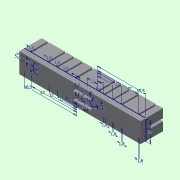
# Autodesk Inventor part: Distance_test_rig
Saved by Autodesk Inventor 2015 (Build 190159000, 159)
## iProperties
Created: 2015-05-18
Part Number: Distance_test_rig
Material: Generic
Document SubType Name: Modeling
Designer: Openlab
Density: 1 g/cm^3
Appearance: Default
Author: Openlab
Autodesk Inventor part; units mm, degrees
ref_plane "YZ Plane" through (0, 0, 0) normal (1, 0, 0) x (0, 1, 0)
ref_plane "XZ Plane" through (0, 0, 0) normal (0, 1, 0) x (-1, 0, 0)
ref_plane "XY Plane" through (0, 0, 0) normal (0, 0, 1) x (1, 0, 0)
sketch "Sketch1" plane through (0, 0, 0) normal (0, 1, 0) x (-1, 0, 0)
  line L0 (73.75, -5.25) -> (61.25, -5.25)
  line L1 (61.25, -5.25) -> (61.25, -17.75)
  line L2 (61.25, -17.75) -> (73.75, -17.75)
  line L3 (73.75, -17.75) -> (73.75, -5.25)
  line L4 (140, 0) -> (0, 0)
  line L5 (0, 0) -> (0, -23)
  line L6 (0, -23) -> (140, -23)
  line L7 (140, -23) -> (140, 0)
  line L8 (77.3838, -11.5) -> (49.3838, -11.5) construction
  line L9 (67.5, -2.25) -> (67.5, -23.25) construction
  line L10 (81.5, -8.9) -> (140, -8.9)
  line L11 (140, -14.1) -> (81.5, -14.1)
  line L12 (48.5, -23) -> (48.5, 0)
  line L13 (46.7, 0) -> (46.7, -23)
  line L14 (38.5, 0) -> (38.5, -23)
  line L15 (36.7, 0) -> (36.7, -23)
  line L16 (28.5, 0) -> (28.5, -23)
  line L17 (26.7, 0) -> (26.7, -23)
  line L18 (8.5, 0) -> (8.5, -23)
  line L19 (6.7, -23) -> (6.7, 0)
  line L20 (53, -10) -> (0, -10)
  line L21 (53, -13) -> (0, -13)
  line L22 (91.5, -14.55) -> (90, -14.55)
  line L23 (90, -14.55) -> (90, -8.45)
  line L24 (90, -8.45) -> (91.5, -8.45)
  line L25 (101.5, -14.55) -> (100, -14.55)
  line L26 (100, -14.55) -> (100, -8.45)
  line L27 (100, -8.45) -> (101.5, -8.45)
  line L28 (111.5, -14.55) -> (110, -14.55)
  line L29 (110, -14.55) -> (110, -8.45)
  line L30 (110, -8.45) -> (111.5, -8.45)
  line L31 (131.5, -14.55) -> (130, -14.55)
  line L32 (130, -14.55) -> (130, -8.45)
  line L33 (130, -8.45) -> (131.5, -8.45)
  line L34 (79.5, 0) -> (79.5, -23)
  line L35 (81.5, -23) -> (81.5, 0)
  line L36 (55.5, 0) -> (55.5, -23)
  line L37 (79.5, -13) -> (73.75, -13)
  line L38 (73.75, -10) -> (79.5, -10)
  line L39 (61.25, -13) -> (55.5, -13)
  line L40 (55.5, -10) -> (61.25, -10)
  line L41 (73.75, -17.75) -> (77.95, -17.75)
  line L42 (77.95, -17.75) -> (77.95, -14.55)
  line L43 (77.95, -14.55) -> (73.75, -14.55)
  line L44 (73.75, -14.55) -> (61.25, -14.55)
  line L45 (56.65, -14.55) -> (56.65, -17.75)
  line L46 (56.65, -17.75) -> (59.85, -17.75)
  line L47 (59.85, -14.55) -> (56.65, -14.55)
  line L48 (59.85, -5.25) -> (56.65, -5.25)
  line L49 (56.65, -5.25) -> (56.65, -8.45)
  line L50 (56.65, -8.45) -> (59.85, -8.45)
  line L51 (61.25, -8.45) -> (73.75, -8.45)
  line L52 (77.95, -8.45) -> (77.95, -5.25)
  line L53 (73.75, -5.25) -> (77.95, -5.25)
  line L54 (77.95, -8.45) -> (73.75, -8.45)
  line L55 (59.85, -17.75) -> (59.85, -14.55)
  line L56 (59.85, -8.45) -> (59.85, -5.25)
  line L57 (61.25, -17.75) -> (59.85, -17.75)
  line L58 (61.25, -14.55) -> (59.85, -14.55)
  line L59 (61.25, -8.45) -> (59.85, -8.45)
  line L60 (61.25, -5.25) -> (59.85, -5.25)
  line L61 (53.5, -14) -> (53, -14)
  line L62 (53, -14) -> (53, -9)
  line L63 (53, -9) -> (53.5, -9)
  line L64 (53.5, -23) -> (53.5, -14)
  line L65 (53.5, -9) -> (53.5, 0)
  line L66 (131.5, -17.5) -> (129.5, -17.5)
  line L67 (129.5, -17.5) -> (129.5, -15.5)
  line L68 (129.5, -15.5) -> (131.5, -15.5)
  line L69 (131.5, -7.5) -> (129.5, -7.5)
  line L70 (129.5, -7.5) -> (129.5, -5.5)
  line L71 (129.5, -5.5) -> (131.5, -5.5)
  line L72 (137, -16.5) -> (85, -16.5) construction
  line L73 (137, -6.5) -> (84.6621, -6.5) construction
  line L74 (133.3, -17.5) -> (135.3, -17.5)
  line L75 (135.3, -17.5) -> (135.3, -15.5)
  line L76 (135.3, -15.5) -> (133.3, -15.5)
  line L77 (133.3, -7.5) -> (135.3, -7.5)
  line L78 (135.3, -7.5) -> (135.3, -5.5)
  line L79 (135.3, -5.5) -> (133.3, -5.5)
  line L80 (133.3, -23) -> (133.3, -17.5)
  line L81 (131.5, -17.5) -> (131.5, -23)
  line L82 (133.3, -15.5) -> (133.3, -7.5)
  line L83 (133.3, -5.5) -> (133.3, 0)
  line L84 (131.5, 0) -> (131.5, -5.5)
  line L85 (131.5, -7.5) -> (131.5, -15.5)
  line L86 (111.5, -15.5) -> (109.5, -15.5)
  line L87 (109.5, -15.5) -> (109.5, -17.5)
  line L88 (115.3, -17.5) -> (115.3, -15.5)
  line L89 (115.3, -15.5) -> (113.3, -15.5)
  line L90 (113.3, -5.5) -> (115.3, -5.5)
  line L91 (115.3, -5.5) -> (115.3, -7.5)
  line L92 (115.3, -7.5) -> (113.3, -7.5)
  line L93 (109.5, -7.5) -> (109.5, -5.5)
  line L94 (109.5, -7.5) -> (111.5, -7.5)
  line L95 (109.5, -5.5) -> (111.5, -5.5)
  line L96 (109.5, -17.5) -> (111.5, -17.5)
  line L97 (113.3, -17.5) -> (115.3, -17.5)
  line L98 (113.3, -17.5) -> (113.3, -23)
  line L99 (111.5, -17.5) -> (111.5, -23)
  line L100 (113.3, 0) -> (113.3, -5.5)
  line L101 (113.3, -7.5) -> (113.3, -15.5)
  line L102 (111.5, 0) -> (111.5, -5.5)
  line L103 (111.5, -7.5) -> (111.5, -15.5)
  line L104 (99.5, -17.5) -> (99.5, -15.5)
  line L105 (105.3, -15.5) -> (105.3, -17.5)
  line L106 (105.3, -17.5) -> (103.3, -17.5)
  line L107 (101.5, -17.5) -> (99.5, -17.5)
  line L108 (99.5, -15.5) -> (101.5, -15.5)
  line L109 (103.3, -15.5) -> (105.3, -15.5)
  line L110 (103.3, -7.5) -> (105.3, -7.5)
  line L111 (105.3, -7.5) -> (105.3, -5.5)
  line L112 (105.3, -5.5) -> (103.3, -5.5)
  line L113 (101.5, -7.5) -> (99.5, -7.5)
  line L114 (99.5, -7.5) -> (99.5, -5.5)
  line L115 (99.5, -5.5) -> (101.5, -5.5)
  line L116 (103.3, -23) -> (103.3, -17.5)
  line L117 (101.5, -17.5) -> (101.5, -23)
  line L118 (103.3, -15.5) -> (103.3, -7.5)
  line L119 (103.3, -5.5) -> (103.3, 0)
  line L120 (101.5, 0) -> (101.5, -5.5)
  line L121 (101.5, -7.5) -> (101.5, -15.5)
  line L122 (91.5, -15.5) -> (89.5, -15.5)
  line L123 (89.5, -15.5) -> (89.5, -17.5)
  line L124 (89.5, -17.5) -> (91.5, -17.5)
  line L125 (93.3, -17.5) -> (95.3, -17.5)
  line L126 (95.3, -17.5) -> (95.3, -15.5)
  line L127 (95.3, -15.5) -> (93.3, -15.5)
  line L128 (93.3, -7.5) -> (95.3, -7.5)
  line L129 (95.3, -7.5) -> (95.3, -5.5)
  line L130 (95.3, -5.5) -> (93.3, -5.5)
  line L131 (91.5, -5.5) -> (89.5, -5.5)
  line L132 (89.5, -5.5) -> (89.5, -7.5)
  line L133 (91.5, -7.5) -> (89.5, -7.5)
  line L134 (93.3, -23) -> (93.3, -17.5)
  line L135 (91.5, -17.5) -> (91.5, -23)
  line L136 (93.3, -15.5) -> (93.3, -7.5)
  line L137 (93.3, -5.5) -> (93.3, 0)
  line L138 (91.5, 0) -> (91.5, -5.5)
  line L139 (91.5, -7.5) -> (91.5, -15.5)
  point P0 (133.3, -8.9)
  point P1 (133.3, -14.1)
  point P2 (131.5, -8.9)
  point P3 (131.5, -14.1)
  point P4 (113.3, -8.9)
  point P5 (111.5, -8.9)
  point P6 (113.3, -14.1)
  point P7 (111.5, -14.1)
  point P8 (103.3, -8.9)
  point P9 (101.5, -8.9)
  point P10 (103.3, -14.1)
  point P11 (101.5, -14.1)
  point P12 (93.3, -8.9)
  point P13 (91.5, -8.9)
  point P14 (93.3, -14.1)
  point P15 (91.5, -14.1)
  point P16 (48.5, -10)
  point P17 (46.7, -10)
  point P18 (48.5, -13)
  point P19 (46.7, -13)
  point P20 (38.5, -13)
  point P21 (36.7, -13)
  point P22 (36.7, -10)
  point P23 (38.5, -10)
  point P24 (28.5, -10)
  point P25 (26.7, -10)
  point P26 (26.7, -13)
  point P27 (28.5, -13)
  point P28 (8.5, -13)
  point P29 (6.7, -13)
  point P30 (6.7, -10)
  point P31 (8.5, -10)
  point P32 (67.5, -11.5)
  point P33 (90, -14.1)
  point P34 (90, -8.9)
  point P35 (130, -14.1)
  point P36 (130, -8.9)
  point P37 (110, -14.1)
  point P38 (110, -8.9)
  point P39 (100, -8.9)
  point P40 (100, -14.1)
  dimension "d12" = 5.2
  dimension "d25" = 3
  dimension "d0" = 12.5
  dimension "d1" = 12.5
  dimension "d3" = 23
  dimension "d18" = 1.8
  dimension "d20" = 1.8
  dimension "d22" = 1.8
  dimension "d24" = 1.8
  dimension "d36" = 6.1
  dimension "d37" = 1.5
  dimension "d43" = 2
  dimension "d52" = 12
  dimension "d57" = 12
  dimension "d62" = 3
  dimension "d63" = 3
  dimension "d70" = 60.5
  dimension "d71" = 7
  dimension "d72" = 17
  dimension "d73" = 27
  dimension "d74" = 47
  dimension "d75" = 55.5
  dimension "d76" = 4.2
  dimension "d77" = 3.2
  dimension "d78" = 3.2
  dimension "d79" = 1.4
  dimension "d80" = 3.2
  dimension "d91" = 5
  dimension "d92" = 0.5
  dimension "d93" = 2
  dimension "d94" = 2
  dimension "d95" = 2
  dimension "d96" = 10
  dimension "d97" = 1.8
  dimension "d98" = 52
  dimension "d99" = 1.8
  dimension "d100" = 32
  dimension "d101" = 1.8
  dimension "d102" = 22
  dimension "d103" = 1.8
  dimension "d104" = 12
  constraints: 268 end point, 117 point on line, 72 perpendicular, 44 vertical, 24 collinear, 20 horizontal, 19 equal length, 13 parallel, 1 coincident, 115 other
  measures "d0" distance of L2.end L1.end
  measures "d1" distance of L0.end L1.end
  measures "d3" distance of L5.end L5.start
  measures "d18" distance between parallel lines of L13 L12
  measures "d20" distance between parallel lines of L15 L14
  measures "d22" distance between parallel lines of L17 L16
  measures "d24" distance between parallel lines of L19 L18
  measures "d36" distance of L31.end L32.end
  measures "d37" distance of L31.start L31.end
  measures "d43" distance between parallel lines of L35 L34
  measures "d52" distance between parallel lines of L36 L9
  measures "d57" distance between parallel lines of L34 L9
  measures "d62" distance between parallel lines of L38 L37
  measures "d63" distance between parallel lines of L40 L39
  measures "d70" distance between parallel lines of L7 L34
  measures "d71" distance between parallel lines of L12 L36
  measures "d72" distance between parallel lines of L14 L36
  measures "d73" distance between parallel lines of L16 L36
  measures "d74" distance between parallel lines of L18 L36
  measures "d75" distance between parallel lines of L5 L36
  measures "d76" distance of L2.end L41.end
  measures "d77" distance of L41.end L42.end
  measures "d78" distance of L52.start L52.end
  measures "d79" distance between parallel lines of L55 L1
  measures "d80" distance of L45.end L46.end
  measures "d91" distance of L61.end L62.end
  measures "d92" distance of L61.start L61.end
  measures "d93" distance between parallel lines of L65 L36
  measures "d94" distance of L66.end L67.end
  measures "d95" distance of L66.start L66.end
  measures "d96" distance between parallel lines of L73 L72
  measures "d97" distance between parallel lines of L84 L83
  measures "d98" distance between parallel lines of L34 L81
  measures "d99" distance between parallel lines of L102 L100
  measures "d100" distance between parallel lines of L99 L34
  measures "d101" distance between parallel lines of L120 L119
  measures "d102" distance between parallel lines of L34 L117
  measures "d103" distance between parallel lines of L138 L137
  measures "d104" distance between parallel lines of L135 L34
extrude "Extrusion10" add sketch "Sketch1" against normal blind 6 contours L0 L60 L48 L49 L50 L59 L1 L40 L36 L4 L34 L38 L3 L54 L52 L53 | L3 L44 L1 L51 | L38 L34 L37 L3 | L1 L39 L36 L40 | L37 L34 L6 L36 L39 L1 L58 L47 L45 L46 L57 L2 L41 L42 L43 L3 | L34 L4 L35 L6 | L36 L6 L64 L61 L62 L63 L65 L4 | L4 L138 L131 L132 L133 L139 L24 L23 L10 L35 | L65 L63 L62 L20 L12 L4 | L35 L11 L23 L22 L139 L122 L123 L124 L135 L6 | L4 L137 L130 L129 L128 L136 L10 L139 L133 L132 L131 L138 | L10 L23 L11 L35 | L6 L12 L21 L62 L61 L64 | L12 L20 L13 L4 | L135 L124 L123 L122 L139 L11 L136 L127 L126 L125 L134 L6 | L4 L120 L115 L114 L113 L121 L27 L26 L10 L136 L128 L129 L130 L137 | L23 L24 L139 L10 | L10 L139 L11 L23 | L6 L13 L21 L12 | L13 L20 L14 L4 | L20 L62 L21 L12 | L12 L21 L13 L20 | L134 L125 L126 L127 L136 L11 L26 L25 L121 L108 L104 L107 L117 L6 | L11 L139 L22 L23 | L4 L119 L112 L111 L110 L118 L10 L121 L113 L114 L115 L120 | L10 L136 L11 L139 | L6 L14 L21 L13 | L14 L20 L15 L4 | L13 L21 L14 L20 | L117 L107 L104 L108 L121 L11 L118 L109 L105 L106 L116 L6 | L4 L102 L95 L93 L94 L103 L30 L29 L10 L118 L110 L111 L112 L119 | L10 L26 L11 L136 | L6 L15 L21 L14 | L15 L20 L16 L4 | L14 L21 L15 L20 | L116 L106 L105 L109 L118 L11 L29 L28 L103 L86 L87 L96 L99 L6 | L4 L100 L90 L91 L92 L101 L10 L103 L94 L93 L95 L102 | L26 L27 L121 L10 | L10 L121 L11 L26 | L6 L16 L21 L15 | L16 L20 L17 L4 | L15 L21 L16 L20 | L99 L96 L87 L86 L103 L11 L101 L89 L88 L97 L98 L6 | L11 L121 L25 L26 | L4 L84 L71 L70 L69 L85 L33 L32 L10 L101 L92 L91 L90 L100 | L10 L118 L11 L121 | L6 L17 L21 L16 | L17 L20 L18 L4 | L16 L21 L17 L20 | L98 L97 L88 L89 L101 L11 L32 L31 L85 L68 L67 L66 L81 L6 | L4 L83 L79 L78 L77 L82 L10 L85 L69 L70 L71 L84 | L10 L29 L11 L118 | L6 L18 L21 L17 | L18 L20 L19 L4 | L17 L21 L18 L20 | L81 L66 L67 L68 L85 L11 L82 L76 L75 L74 L80 L6 | L4 L7 L10 L82 L77 L78 L79 L83 | L29 L30 L103 L10 | L10 L103 L11 L29 | L6 L19 L21 L18 | L19 L20 L5 L4 | L18 L21 L19 L20 | L80 L74 L75 L76 L82 L11 L7 L6 | L11 L103 L28 L29 | L10 L101 L11 L103 | L6 L5 L21 L19 | L19 L21 L5 L20 | L7 L11 L82 L10 | L10 L32 L11 L101 | L82 L11 L85 L10 | L32 L33 L85 L10 | L10 L85 L11 L32 | L11 L85 L31 L32
extrude "Extrusion11" add sketch "Sketch1" against normal blind 3 contours L3 L51 L1 L0 | L1 L59 L56 L60 | L3 L2 L1 L44 | L1 L57 L55 L58
extrude "Extrusion12" add sketch "Sketch1" along normal blind 5 contours L0 L60 L48 L49 L50 L59 L1 L40 L36 L4 L34 L38 L3 L54 L52 L53 | L1 L59 L56 L60 | L38 L34 L37 L3 | L1 L39 L36 L40 | L37 L34 L6 L36 L39 L1 L58 L47 L45 L46 L57 L2 L41 L42 L43 L3 | L1 L57 L55 L58 | L4 L138 L131 L132 L133 L139 L24 L23 L10 L35 | L65 L63 L62 L20 L12 L4 | L35 L11 L23 L22 L139 L122 L123 L124 L135 L6 | L10 L23 L11 L35 | L6 L12 L21 L62 L61 L64 | L4 L120 L115 L114 L113 L121 L27 L26 L10 L136 L128 L129 L130 L137 | L13 L20 L14 L4 | L20 L62 L21 L12 | L134 L125 L126 L127 L136 L11 L26 L25 L121 L108 L104 L107 L117 L6 | L6 L14 L21 L13 | L13 L21 L14 L20 | L4 L102 L95 L93 L94 L103 L30 L29 L10 L118 L110 L111 L112 L119 | L10 L26 L11 L136 | L15 L20 L16 L4 | L116 L106 L105 L109 L118 L11 L29 L28 L103 L86 L87 L96 L99 L6 | L6 L16 L21 L15 | L15 L21 L16 L20 | L4 L84 L71 L70 L69 L85 L33 L32 L10 L101 L92 L91 L90 L100 | L17 L20 L18 L4 | L98 L97 L88 L89 L101 L11 L32 L31 L85 L68 L67 L66 L81 L6 | L10 L29 L11 L118 | L6 L18 L21 L17 | L17 L21 L18 L20 | L4 L7 L10 L82 L77 L78 L79 L83 | L19 L20 L5 L4 | L80 L74 L75 L76 L82 L11 L7 L6 | L6 L5 L21 L19 | L19 L21 L5 L20 | L7 L11 L82 L10 | L10 L32 L11 L101
extrude "Extrusion13" add sketch "Sketch1" along normal blind 20 contours L0 L60 L48 L49 L50 L59 L1 L40 L36 L4 L34 L38 L3 L54 L52 L53 | L1 L59 L56 L60 | L37 L34 L6 L36 L39 L1 L58 L47 L45 L46 L57 L2 L41 L42 L43 L3 | L1 L57 L55 L58 | L4 L138 L131 L132 L133 L139 L24 L23 L10 L35 | L65 L63 L62 L20 L12 L4 | L35 L11 L23 L22 L139 L122 L123 L124 L135 L6 | L6 L12 L21 L62 L61 L64 | L4 L120 L115 L114 L113 L121 L27 L26 L10 L136 L128 L129 L130 L137 | L13 L20 L14 L4 | L134 L125 L126 L127 L136 L11 L26 L25 L121 L108 L104 L107 L117 L6 | L6 L14 L21 L13 | L4 L102 L95 L93 L94 L103 L30 L29 L10 L118 L110 L111 L112 L119 | L15 L20 L16 L4 | L116 L106 L105 L109 L118 L11 L29 L28 L103 L86 L87 L96 L99 L6 | L6 L16 L21 L15 | L4 L84 L71 L70 L69 L85 L33 L32 L10 L101 L92 L91 L90 L100 | L17 L20 L18 L4 | L98 L97 L88 L89 L101 L11 L32 L31 L85 L68 L67 L66 L81 L6 | L6 L18 L21 L17 | L4 L7 L10 L82 L77 L78 L79 L83 | L19 L20 L5 L4 | L80 L74 L75 L76 L82 L11 L7 L6 | L6 L5 L21 L19
extrude "Extrusion14" add sketch "Sketch1" along normal blind 2.5 contours L3 L51 L1 L0 | L3 L44 L1 L51 | L3 L2 L1 L44
body "Solid3"
